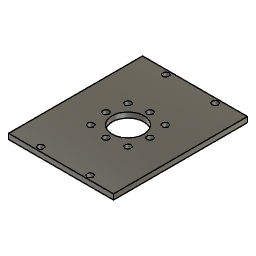
Motor_Mount_LIVE (Autodesk Fusion 360 design; units mm, degrees)
Autodesk Fusion 360 part; units mm, degrees
sketch "Sketch1" plane through (0, 0, 0) normal (0, 0, 1) x (1, 0, 0)
  circle A0 centre (0, 0) radius 29.75
  circle A1 centre (0, 0) radius 12.5
  circle A2 centre (0, 0) radius 15
  circle A3 centre (0, 12.5) radius 1.7
  circle A4 centre (-10.6066, 10.6066) radius 1.7
  circle A5 centre (-10.6066, -10.6066) radius 1.7
  circle A6 centre (-12.5, 0) radius 1.7
  circle A7 centre (10.6066, -10.6066) radius 1.7
  circle A8 centre (0, -12.5) radius 1.7
  circle A9 centre (10.6066, 10.6066) radius 1.7
  circle A10 centre (12.5, 0) radius 1.7
  circle A11 centre (-14, 35.5) radius 1.7
  circle A12 centre (14, 35.5) radius 1.7
  circle A13 centre (14, -35.5) radius 1.7
  circle A14 centre (-14, -35.5) radius 1.7
  line L0 (-29.75, 38) -> (29.75, 38)
  line L1 (29.75, 38) -> (29.75, -38)
  line L2 (29.75, -38) -> (-29.75, -38)
  line L3 (-29.75, -38) -> (-29.75, 38)
  circle A15 centre (0, 0) radius 9
  dimension "d1" = 59.5
  dimension "d2" = 25
  dimension "d3" = 30
  dimension "d5" = 3.4
  dimension "d10" = 360
  dimension "d13" = 3.4
  dimension "d14" = 3.4
  dimension "d15" = 3.4
  dimension "d16" = 3.4
  dimension "d17" = 59.5
  dimension "d18" = 76
  dimension "d19" = 18
  constraint coincident A0.centre A1.centre
  constraint horizontal L0
  constraint vertical L1
  constraint horizontal L2
  constraint vertical L3
  measures "d1" diameter of A0
  measures "d2" diameter of A1
  measures "d3" diameter of A2
  measures "d5" diameter of A3
  measures "d13" diameter of A11
  measures "d14" diameter of A12
  measures "d15" diameter of A14
  measures "d16" diameter of A13
  measures "d17" distance of L0.start L0.end
  measures "d18" distance of L0.start L2.end
  measures "d19" diameter of A15
extrude "Extrude1" add sketch "Sketch1" along normal blind 3 contours A0 | A0 L1 L2 L3 | A0 L0 L1 L3 | A1 A3 A6 A8 A10 | A2 A4 A5 A7 A9
